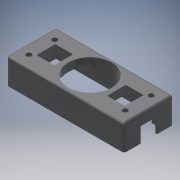
# Autodesk Inventor part: Accelite_Controller_cover_new
Saved by Autodesk Inventor 2018 (Build 220112000, 112)
## iProperties
Created: 2014-07-12
Part Number: Accelite_Controller_cover_new
Material: ABS プラスチック
Document SubType Name: Modeling
Designer: andou
Density: 1.06 g/cm^3
Appearance: 滑らか - 標準の灰色
Mass: 3.87174 g
Surface Area: 42.7791 cm^2
Volume: 3.65258 cm^3
Author: andou
Autodesk Inventor part; units mm, degrees
ref_plane "YZ Plane" through (0, 0, 0) normal (1, 0, 0) x (0, 1, 0)
ref_plane "XZ Plane" through (0, 0, 0) normal (0, 1, 0) x (-1, 0, 0)
ref_plane "XY Plane" through (0, 0, 0) normal (0, 0, 1) x (1, 0, 0)
sketch "スケッチ1" plane through (0, 0, 0) normal (0, 0, 1) x (1, 0, 0)
  line L0 (25, -10.5) -> (-25, -10.5)
  line L1 (-25, -10.5) -> (-25, 10.5)
  line L2 (-25, 10.5) -> (25, 10.5)
  line L3 (25, 10.5) -> (25, -10.5)
  line L4 (25, -10.5) -> (-25, 10.5) construction
  line L5 (-25, -10.5) -> (25, 10.5) construction
  point P0 (0, 0)
  dimension "d0" = 50
  dimension "d2" = 21
  constraints: 12 end point, 2 midpoint, 2 parallel, 1 horizontal, 1 perpendicular
  measures "d0" distance of L1.end L2.end
  measures "d2" distance of L0.end L1.end
extrude "押し出し1" add sketch "スケッチ1" along normal blind 11
sketch "スケッチ2" plane through (0, 0, 11) normal (0, 0, 1) x (1, 0, 0)
  line L0 (25, -10.5) -> (25, 10.5) projected
  circle A0 centre (0, 0) radius 9
  dimension "d5" = 18
  dimension "d9" = 0
  dimension "d10" = 25
  constraints: 1 centre point
  measures "d5" diameter of A0
  measures "d9" distance of A0.centre point (0, 0)
  measures "d10" distance from line of L0 A0.centre
hole "穴1" at (0, 0, 11) direction (0, 0, -1) diameter 18.5 end through all
sketch "スケッチ3" plane through (0, 0, 11) normal (0, 0, 1) x (1, 0, 0)
  circle A0 centre (0, 0) radius 9.25 projected
  line L0 (-18.75, 4) -> (-11.25, 4)
  line L1 (-11.25, 4) -> (-11.25, -4)
  line L2 (-11.25, -4) -> (-18.75, -4)
  line L3 (-18.75, -4) -> (-18.75, 4)
  line L4 (11.25, 4) -> (18.75, 4)
  line L5 (18.75, 4) -> (18.75, -4)
  line L6 (18.75, -4) -> (11.25, -4)
  line L7 (11.25, -4) -> (11.25, 4)
  line L8 (-11.25, -4) -> (-18.75, -4)
  line L9 (-18.75, -4) -> (-18.75, 4)
  line L10 (-18.75, 4) -> (-11.25, 4)
  line L11 (-11.25, 4) -> (-11.25, -4)
  line L12 (-11.25, -4) -> (-18.75, 4) construction
  line L13 (-18.75, -4) -> (-11.25, 4) construction
  line L14 (18.75, -4) -> (11.25, -4)
  line L15 (11.25, -4) -> (11.25, 4)
  line L16 (11.25, 4) -> (18.75, 4)
  line L17 (18.75, 4) -> (18.75, -4)
  line L18 (18.75, -4) -> (11.25, 4) construction
  line L19 (11.25, -4) -> (18.75, 4) construction
  point P0 (-15, 0)
  point P1 (15, 0)
  dimension "d19" = 7.5
  dimension "d21" = 8
  dimension "d122" = 15
  dimension "d123" = 15
  dimension "d124" = 0
  dimension "d125" = 0
  constraints: 40 end point, 8 parallel, 4 horizontal, 4 midpoint, 4 perpendicular, 2 equal length
  measures "d19" distance of L0.start L0.end
  measures "d21" distance of L4.end L5.end
  measures "d122" distance of A0.centre point (-15, 0)
  measures "d123" distance of point (15, 0) A0.centre
  measures "d124" vertical distance of A0.centre point (-15, 0)
  measures "d125" vertical distance of point (15, 0) A0.centre
extrude "押し出し2" cut sketch "スケッチ3" against normal blind 11 contours L0 L1 L2 L3 | L4 L5 L6 L7
sketch "スケッチ4" plane through (0, 0, 11) normal (0, 0, 1) x (1, 0, 0)
  circle A0 centre (0, 0) radius 9.25 projected
  line L0 (25, 10.5) -> (-25, 10.5) projected
  line L1 (-25, 10.5) -> (-25, -10.5) projected
  circle A1 centre (-20.5, 5.5) radius 1.1
  line L2 (0, 0) -> (0, 10.5)
  line L3 (0, 0) -> (-25, 0)
  circle A2 centre (-20.5, -5.5) radius 1.1
  circle A3 centre (20.5, -5.5) radius 1.1
  circle A4 centre (20.5, 5.5) radius 1.1
  dimension "d26" = 2.2
  dimension "d28" = 20.5
  dimension "d29" = 5.5
  dimension "d32" = 41
  dimension "d35" = 11
  constraints: 4 centre point, 4 end point, 3 coincident, 3 equal radius, 2 midpoint, 1 horizontal, 1 perpendicular, 1 vertical, 3 other
  measures "d26" diameter of A1
  measures "d28" horizontal distance of L2.start A1.centre
  measures "d29" vertical distance of A1.centre L2.start
  measures "d32" distance of A1.centre point (20.5, 5.5)
  measures "d35" distance of A1.centre point (-20.5, -5.5)
hole "穴2" at (-20.5, 5.5, 11) at (-20.5, -5.5, 11) at (20.5, -5.5, 11) at (20.5, 5.5, 11) direction (0, 0, -1) diameter 2.2 end through all
sketch "スケッチ5" plane through (0, 0, 0) normal (0, 0, -1) x (-1, 0, 0)
  circle A0 centre (-20.5, -5.5) radius 1.1 projected
  circle A1 centre (20.5, 5.5) radius 1.1 projected
  circle A2 centre (20.5, -5.5) radius 1.1 projected
  circle A3 centre (-20.5, 5.5) radius 1.1 projected
  line L0 (18.75, 4) -> (18.75, -4) projected
  line L1 (18.75, -4) -> (11.25, -4) projected
  line L2 (11.25, -4) -> (11.25, 4) projected
  line L3 (11.25, 4) -> (18.75, 4) projected
  line L4 (-11.25, 4) -> (-11.25, -4) projected
  line L5 (-11.25, -4) -> (-18.75, -4) projected
  line L6 (-18.75, -4) -> (-18.75, 4) projected
  line L7 (-18.75, 4) -> (-11.25, 4) projected
  circle A4 centre (0, 0) radius 9.25 projected
  line L8 (22.75, -7.75) -> (-22.75, -7.75)
  line L9 (-22.75, -7.75) -> (-22.75, 7.75)
  line L10 (-22.75, 7.75) -> (22.75, 7.75)
  line L11 (22.75, 7.75) -> (22.75, -7.75)
  line L12 (22.75, -7.75) -> (-22.75, 7.75) construction
  line L13 (-22.75, -7.75) -> (22.75, 7.75) construction
  dimension "d45" = 45.5
  dimension "d47" = 15.5
  constraints: 12 end point, 2 midpoint, 2 parallel, 1 horizontal, 1 perpendicular
  measures "d45" distance of L9.end L10.end
  measures "d47" distance of L10.end L8.start
extrude "押し出し3" cut sketch "スケッチ5" against normal blind 7.5 contours A4 L8 L10 | A4 L10 L11 L8 | A4 L8 L9 L10
sketch "スケッチ11" plane through (0, 0, 0) normal (0, 0, -1) x (-1, 0, 0)
  line L0 (-22.75, 7.75) -> (-5.0498, 7.75) projected
  arc A0 (5.0498, 7.75) -> (-5.0498, 7.75) centre (0, 0) ccw projected
  line L1 (5.0498, 7.75) -> (22.75, 7.75) projected
  line L2 (22.75, 7.75) -> (22.75, -7.75) projected
  line L3 (22.75, -7.75) -> (5.0498, -7.75) projected
  arc A1 (-5.0498, -7.75) -> (5.0498, -7.75) centre (0, 0) ccw projected
  line L4 (-5.0498, -7.75) -> (-22.75, -7.75) projected
  line L5 (-22.75, -7.75) -> (-22.75, 7.75) projected
  line L6 (-24.25, 9.75) -> (24.25, 9.75)
  line L7 (24.25, 9.75) -> (24.25, -9.75)
  line L8 (24.25, -9.75) -> (-24.25, -9.75)
  line L9 (-24.25, -9.75) -> (-24.25, 9.75)
  line L10 (24.25, -9.75) -> (-24.25, -9.75)
  line L11 (-24.25, -9.75) -> (-24.25, 9.75)
  line L12 (-24.25, 9.75) -> (24.25, 9.75)
  line L13 (24.25, 9.75) -> (24.25, -9.75)
  line L14 (24.25, -9.75) -> (-24.25, 9.75) construction
  line L15 (-24.25, -9.75) -> (24.25, 9.75) construction
  dimension "d89" = 19.5
  dimension "d126" = 48.5
  dimension "d128" = 0
  dimension "d129" = 0
  constraints: 20 end point, 4 parallel, 2 horizontal, 2 midpoint, 2 perpendicular
  measures "d89" distance between parallel lines of L8 L6
  measures "d126" distance of L6.start L6.end
  measures "d128" distance between parallel lines of L7 L13
  measures "d129" distance between parallel lines of L8 L10
extrude "押し出し9" cut sketch "スケッチ11" against normal blind 3
sketch "スケッチ13" plane through (0, 0, 0) normal (0, 0, -1) x (-1, 0, 0)
  line L0 (-25, 10.5) -> (-25, -10.5) projected
  line L1 (-25, 3.5) -> (-22.5, 3.5)
  line L2 (-22.5, 3.5) -> (-22.5, -3.5)
  line L3 (-22.5, -3.5) -> (-25, -3.5)
  line L4 (-25, -3.5) -> (-25, 3.5)
  point P0 (0, 0)
  dimension "d96" = 7
  dimension "d99" = 2.5
  dimension "d119" = 3.5
  constraints: 8 end point, 2 parallel, 1 horizontal, 1 perpendicular, 1 point on line
  measures "d96" distance of L1.end L2.end
  measures "d99" distance between parallel lines of L0 L2
  measures "d119" distance from line of point (0, 0) L3
extrude "押し出し11" cut sketch "スケッチ13" against normal blind 6.4
fillet "フィレット2" radius 1 8 edges at (-25, 0, 11) (0, -10.5, 11) (0, 10.5, 11) (25, 0, 11) (25, -10.5, 5.5) (25, 10.5, 5.5) (-25, 10.5, 5.5) (-25, -10.5, 5.5)
sketch "スケッチ14" plane through (0, 0, 7.5) normal (0, 0, -1) x (-1, 0, 0)
  arc A0 (25, 9.5) -> (24, 10.5) centre (24, 9.5) ccw projected
  line L0 (25, 9.5) -> (25, -9.5) projected
  arc A1 (24, -10.5) -> (25, -9.5) centre (24, -9.5) ccw projected
  line L1 (24, -10.5) -> (-24, -10.5) projected
  arc A2 (-25, -9.5) -> (-24, -10.5) centre (-24, -9.5) ccw projected
  line L2 (-25, -9.5) -> (-25, 9.5) projected
  arc A3 (-24, 10.5) -> (-25, 9.5) centre (-24, 9.5) ccw projected
  line L3 (-24, 10.5) -> (24, 10.5) projected
  line L4 (5.0498, -7.75) -> (22.75, -7.75) projected
  line L5 (22.75, -7.75) -> (22.75, 7.75) projected
  line L6 (22.75, 7.75) -> (5.0498, 7.75) projected
  arc A4 (5.0498, 7.75) -> (-5.0498, 7.75) centre (0, 0) ccw projected
  line L7 (-5.0498, 7.75) -> (-22.75, 7.75) projected
  line L8 (-22.75, 7.75) -> (-22.75, -7.75) projected
  line L9 (-22.75, -7.75) -> (-5.0498, -7.75) projected
  arc A5 (-5.0498, 7.75) -> (-5.0498, -7.75) centre (0, 0) ccw projected
  arc A6 (5.0498, -7.75) -> (5.0498, 7.75) centre (0, 0) ccw projected
  arc A7 (-5.0498, -7.75) -> (5.0498, -7.75) centre (0, 0) ccw projected
  line L10 (-18.75, 4) -> (-18.75, -4) projected
  line L11 (-18.75, -4) -> (-11.25, -4) projected
  line L12 (-11.25, -4) -> (-11.25, 4) projected
  line L13 (-11.25, 4) -> (-18.75, 4) projected
  line L14 (11.25, 4) -> (11.25, -4) projected
  line L15 (11.25, -4) -> (18.75, -4) projected
  line L16 (18.75, -4) -> (18.75, 4) projected
  line L17 (18.75, 4) -> (11.25, 4) projected
  circle A8 centre (-20.5, -5.5) radius 1.1 projected
  circle A9 centre (20.5, 5.5) radius 1.1 projected
  circle A10 centre (20.5, -5.5) radius 1.1 projected
  circle A11 centre (-20.5, 5.5) radius 1.1 projected
  line L18 (-18, 6.5) -> (-12, 6.5)
  line L19 (-12, 6.5) -> (-12, -6.5)
  line L20 (-12, -6.5) -> (-18, -6.5)
  line L21 (-18, -6.5) -> (-18, 6.5)
  line L22 (0, 10.5) -> (0, -10.5)
  line L23 (18, 6.5) -> (12, 6.5)
  line L24 (12, 6.5) -> (12, -6.5)
  line L25 (12, -6.5) -> (18, -6.5)
  line L26 (18, -6.5) -> (18, 6.5)
  point P0 (-18.75, -3.6953)
  point P1 (-18.5202, -4)
  dimension "d103" = 2.5
  dimension "d104" = 2.5
  dimension "d105" = 6
  dimension "d106" = 0.75
  constraints: 18 end point, 4 symmetric about line, 2 midpoint, 2 parallel, 1 horizontal, 1 perpendicular
  measures "d103" distance between parallel lines of L13 L18
  measures "d104" distance between parallel lines of L11 L20
  measures "d105" distance of L18.start L18.end
  measures "d106" distance between parallel lines of L21 L10
extrude "押し出し12" cut sketch "スケッチ14" against normal blind 2.5 contours L21 L18 L19 L13 | L13 L19 L11 L21 | L11 L19 L20 L21 | L24 L23 L26 L17 | L17 L26 L15 L24 | L15 L26 L25 L24
sketch "スケッチ15" plane through (0, 0, 7.5) normal (0, 0, -1) x (-1, 0, 0)
  line L0 (-22.75, -7.75) -> (-22.75, 7.75) projected
  arc A0 (25, 9.5) -> (24, 10.5) centre (24, 9.5) ccw projected
  line L1 (25, 9.5) -> (25, -9.5) projected
  arc A1 (24, -10.5) -> (25, -9.5) centre (24, -9.5) ccw projected
  line L2 (24, -10.5) -> (-24, -10.5) projected
  arc A2 (-25, -9.5) -> (-24, -10.5) centre (-24, -9.5) ccw projected
  line L3 (-25, -9.5) -> (-25, 9.5) projected
  arc A3 (-24, 10.5) -> (-25, 9.5) centre (-24, 9.5) ccw projected
  line L4 (-24, 10.5) -> (24, 10.5) projected
  line L5 (5.0498, -7.75) -> (22.75, -7.75) projected
  line L6 (22.75, -7.75) -> (22.75, 7.75) projected
  line L7 (22.75, 7.75) -> (5.0498, 7.75) projected
  arc A4 (5.0498, 7.75) -> (-5.0498, 7.75) centre (0, 0) ccw projected
  line L8 (-5.0498, 7.75) -> (-22.75, 7.75) projected
  line L9 (-22.75, 7.75) -> (-22.75, -7.75) projected
  line L10 (-22.75, -7.75) -> (-5.0498, -7.75) projected
  arc A5 (-5.0498, 7.75) -> (-5.0498, -7.75) centre (0, 0) ccw projected
  arc A6 (5.0498, -7.75) -> (5.0498, 7.75) centre (0, 0) ccw projected
  arc A7 (-5.0498, -7.75) -> (5.0498, -7.75) centre (0, 0) ccw projected
  line L11 (-18.75, 4) -> (-18.75, -4) projected
  line L12 (-18.75, -4) -> (-18, -4) projected
  line L13 (18.75, -4) -> (18.75, 4) projected
  line L14 (18.75, 4) -> (18, 4) projected
  circle A8 centre (-20.5, -5.5) radius 1.1 projected
  circle A9 centre (20.5, 5.5) radius 1.1 projected
  circle A10 centre (20.5, -5.5) radius 1.1 projected
  circle A11 centre (-20.5, 5.5) radius 1.1 projected
  line L15 (-22.75, 3.5) -> (-18.75, 3.5)
  line L16 (-18.75, 3.5) -> (-18.75, -3.5)
  line L17 (-18.75, -3.5) -> (-22.75, -3.5)
  line L18 (-22.75, -3.5) -> (-22.75, 3.5)
  line L19 (-18, -4) -> (-18, -6.5) projected
  line L20 (-18, -6.5) -> (-12, -6.5) projected
  line L21 (-12, 4) -> (-12, 6.5) projected
  line L22 (-12, 6.5) -> (-18, 6.5) projected
  line L23 (-18, 6.5) -> (-18, 4) projected
  line L24 (0, 10.5) -> (0, -10.5)
  line L25 (18.75, 3.5) -> (22.75, 3.5)
  line L26 (22.75, 3.5) -> (22.75, -3.5)
  line L27 (22.75, -3.5) -> (18.75, -3.5)
  line L28 (18.75, -3.5) -> (18.75, 3.5)
  line L29 (12, -6.5) -> (18, -6.5) projected
  line L30 (18, -6.5) -> (18, -4) projected
  line L31 (18, 4) -> (18, 6.5) projected
  line L32 (18, 6.5) -> (12, 6.5) projected
  line L33 (12, 6.5) -> (12, 4) projected
  line L34 (-12, -6.5) -> (-12, -4) projected
  line L35 (-11.25, -4) -> (-11.25, 4) projected
  line L36 (-11.25, 4) -> (-12, 4) projected
  line L37 (-18, 4) -> (-18.75, 4) projected
  line L38 (11.25, 4) -> (11.25, -4) projected
  line L39 (11.25, -4) -> (12, -4) projected
  line L40 (12, -4) -> (12, -6.5) projected
  line L41 (18, -4) -> (18.75, -4) projected
  line L42 (12, 4) -> (11.25, 4) projected
  line L43 (-12, -4) -> (-11.25, -4) projected
  point P0 (-18.75, -3.6953)
  point P1 (-18.5202, -4)
  dimension "d110" = 7
  dimension "d111" = 4
  dimension "d113" = 7
  dimension "d130" = 3.5
  dimension "d131" = 3.5
  constraints: 18 end point, 4 parallel, 3 point on line, 2 horizontal, 2 midpoint, 2 perpendicular
  measures "d110" distance of L15.end L16.end
  measures "d111" distance between parallel lines of L0 L16
  measures "d113" distance of L27.end L25.start
  measures "d130" distance from line of point (0, 0) L15
  measures "d131" distance from line of L25 point (0, 0)
extrude "押し出し13" cut sketch "スケッチ15" against normal blind 1.5 contours L0 L15 L11 L17 | L27 L13 L25 L6
sketch "スケッチ18" plane through (0, 0, 7.5) normal (0, 0, -1) x (-1, 0, 0)
  arc A0 (5.0498, -7.75) -> (5.0498, 7.75) centre (0, 0) ccw projected
  line L0 (-22.75, 3.5) -> (-18.75, 3.5) projected
  line L1 (-18.75, 4) -> (-18.75, 3.5) projected
  line L2 (-18, 4) -> (-18.75, 4) projected
  line L3 (-18, 4) -> (-18, 6.5) projected
  line L4 (-18, 6.5) -> (-12, 6.5) projected
  line L5 (-12, 6.5) -> (-12, 4) projected
  line L6 (-11.25, 4) -> (-12, 4) projected
  line L7 (-11.25, -4) -> (-11.25, 4) projected
  line L8 (-12, -4) -> (-11.25, -4) projected
  line L9 (-12, -4) -> (-12, -6.5) projected
  line L10 (-12, -6.5) -> (-18, -6.5) projected
  line L11 (-18, -6.5) -> (-18, -4) projected
  line L12 (-18.75, -4) -> (-18, -4) projected
  line L13 (-18.75, -3.5) -> (-18.75, -4) projected
  line L14 (-18.75, -3.5) -> (-22.75, -3.5) projected
  line L15 (-22.75, -7.75) -> (-22.75, -3.5) projected
  line L16 (-5.0498, -7.75) -> (-22.75, -7.75) projected
  arc A1 (-5.0498, 7.75) -> (-5.0498, -7.75) centre (0, 0) ccw projected
  line L17 (-22.75, 7.75) -> (-5.0498, 7.75) projected
  line L18 (-22.75, 3.5) -> (-22.75, 7.75) projected
  circle A2 centre (-20.5, 5.5) radius 1.1 projected
  circle A3 centre (-20.5, -5.5) radius 1.1 projected
  line L19 (10.5, 3.5) -> (-10.5, 3.5)
  line L20 (-10.5, 3.5) -> (-10.5, 6.75)
  line L21 (-10.5, 6.75) -> (10.5, 6.75)
  line L22 (10.5, 6.75) -> (10.5, 3.5)
  line L23 (10.5, 3.5) -> (-10.5, 6.75) construction
  line L24 (-10.5, 3.5) -> (10.5, 6.75) construction
  line L25 (-9.25, 0) -> (9.25, 0)
  line L26 (10.5, -3.5) -> (-10.5, -3.5)
  line L27 (-10.5, -3.5) -> (-10.5, -6.75)
  line L28 (-10.5, -6.75) -> (10.5, -6.75)
  line L29 (10.5, -6.75) -> (10.5, -3.5)
  line L30 (10.5, -3.5) -> (-10.5, -6.75) construction
  line L31 (-10.5, -3.5) -> (10.5, -6.75) construction
  point P0 (0, 5.125)
  point P1 (0, -5.125)
  dimension "d134" = 3.25
  dimension "d135" = 5.125
  dimension "d136" = 0
  dimension "d137" = 21
  constraints: 26 end point, 5 symmetric about line, 4 midpoint, 2 parallel, 2 point on circle, 1 horizontal, 1 perpendicular
  measures "d134" distance of L21.end L19.start
  measures "d135" distance of point (0, 5.125) A0.centre
  measures "d136" horizontal distance of point (0, 5.125) A0.centre
  measures "d137" distance of L20.end L21.end
extrude "押し出し14" cut sketch "スケッチ18" against normal blind 1 contours L28 A1 L26 A0 | A0 L26 L29 L28 | L28 L27 L26 A1 | L19 A1 L21 A0 | A0 L21 L22 L19 | L19 L20 L21 A1
